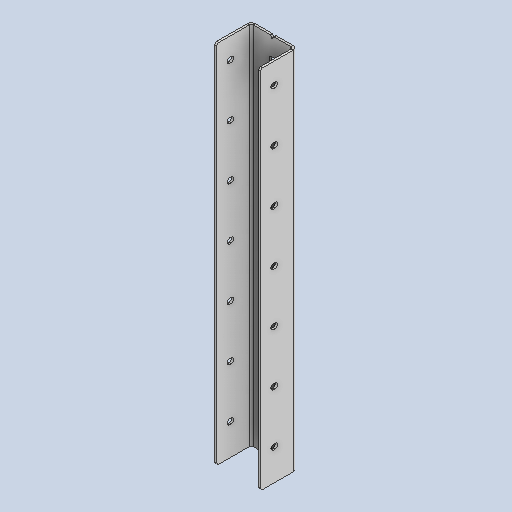
# Autodesk Inventor part: NDM 4.0.1 father bottom
Saved by Autodesk Inventor 2025 (Build 290162010, 162A)
## iProperties
Created: 2023-07-04
Part Number: NDM 4.0.1 father bottom
Material: Stainless Steel
Document SubType Name: Sheet Metal
Designer: user
Density: 8 g/cm^3
Sheet Metal Rule: Default_mm
Appearance: Default
Flat Pattern Width: 10.7048 cm
Flat Pattern Length: 35 cm
Flat Pattern Area: 374.667 cm^2
Sheet Metal Width: 107,048 mm
Sheet Metal Length: 350,000 mm
Sheet Metal Area: 37466,725 mm^2
Stock Number: NDM 7.1 папа ноги домкрат
Description: 2mm
Mass: 592.546 g
Surface Area: 766.755 cm^2
Volume: 74.0682 cm^3
Author: user
Revision Number: 8
Autodesk Inventor part; units mm, degrees
ref_plane "YZ Plane" through (0, 0, 0) normal (1, 0, 0) x (0, 1, 0)
ref_plane "XZ Plane" through (0, 0, 0) normal (0, 1, 0) x (-1, 0, 0)
ref_plane "XY Plane" through (0, 0, 0) normal (0, 0, 1) x (1, 0, 0)
sketch "Sketch1" plane through (0, 0, 0) normal (0, 0, 1) x (1, 0, 0)
  line L0 (-20, 175) -> (20, 175)
  line L1 (20, 175) -> (20, -175)
  line L2 (20, -175) -> (-20, -175)
  line L3 (-20, -175) -> (-20, 175)
  line L4 (-20, 175) -> (20, -175) construction
  line L5 (20, 175) -> (-20, -175) construction
  point P0 (0, 0)
  point P1 (0, 0)
  dimension "d0" = 40
  dimension "d1" = 350
  constraints: 12 end point, 2 midpoint, 1 coincident, 1 horizontal, 1 parallel, 1 perpendicular
  measures "d0" distance of L1.end L2.end
  measures "d1" distance of L2.end L0.start
extrude "Plate1" add sketch "Sketch1" along normal blind 2
sketch "Sketch2" plane through (-20, -175, 2) normal (-1, 0, 0) x (0, -1, 0)
  line L0 (-350, 0) -> (0, 0)
  line L1 (0, 0) -> (0, 33)
  line L2 (0, 33) -> (-350, 33)
  line L3 (-350, 33) -> (-350, 0)
  constraints: 6 end point, 1 horizontal, 1 perpendicular, 1 vertical
edge flange "Flange1" height 35 angle 90 thickness 2 bend radius 2 thickness toward (-1, 0, 0) relief tear relief width 2 relief depth 1 corner gap 2 corner form 0 edges at (-20, 0, 2) (20, 0, 2) wall of the first edge with corners at (-20, 175, 2) (-20, -175, 2) (-20, -175, 35) (-20, 175, 35)
bend "Bend1"
corner "Corner1"
sketch "Sketch3" plane through (0, 0, 0) normal (1, 0, 0) x (0, 1, 0)
  line L0 (-175, 4) -> (175, 4) projected
  line L1 (175, 35) -> (175, 4) projected
  line L2 (-175, 35) -> (175, 35) projected
  line L3 (-175, 4) -> (-175, 35) projected
  circle A0 centre (-145, 22) radius 2.5
  line L4 (-145, 22.75) -> (-145, 21.25) construction
  line L5 (-147.5, 22.75) -> (-147.5, 21.25)
  line L6 (-142.5, 21.25) -> (-142.5, 22.75)
  arc A1 (-142.5, 22.75) -> (-147.5, 22.75) centre (-145, 22.75) ccw
  arc A2 (-147.5, 21.25) -> (-142.5, 21.25) centre (-145, 21.25) ccw
  point P0 (0, 0)
  point P1 (-142.5, 22)
  point P2 (-147.5, 22)
  dimension "d13" = 5
  dimension "d14" = 13
  dimension "d15" = 30
  dimension "d29" = 1.5
  constraints: 8 end point, 5 tangent, 4 point on circle, 3 centre point, 1 coincident, 1 midpoint, 1 parallel, 1 vertical
  measures "d13" diameter of A0
  measures "d14" distance from line of A0.centre L2
  measures "d15" distance from line of L3 A0.centre
  measures "d29" distance of L4.start L4.end
extrude "Extrusion1" cut sketch "Sketch3" along normal through all both and the other way through all contours A0 | L6 A2 L5 A0 | A0 L5 A1 L6
sketch "Sketch4" plane through (0, 0, 0) normal (0, 0, -1) x (-1, 0, 0)
  circle A0 centre (0, -145) radius 2.5
  line L0 (-18, -175) -> (18, -175) projected
  line L1 (-0.5, -145) -> (0.5, -145) construction
  line L2 (-0.5, -147.5) -> (0.5, -147.5)
  line L3 (0.5, -142.5) -> (-0.5, -142.5)
  arc A1 (-0.5, -142.5) -> (-0.5, -147.5) centre (-0.5, -145) ccw
  arc A2 (0.5, -147.5) -> (0.5, -142.5) centre (0.5, -145) ccw
  point P0 (0, 0)
  point P1 (0, -175)
  point P2 (18, -175)
  point P3 (0, -142.5)
  point P4 (0, -147.5)
  dimension "d21" = 5
  dimension "d22" = 30
  dimension "d28" = 1
  constraints: 8 end point, 5 tangent, 4 point on circle, 3 centre point, 1 coincident, 1 horizontal, 1 midpoint, 1 parallel, 1 vertical alignment, 2 other
  measures "d21" diameter of A0
  measures "d28" distance of L1.start L1.end
extrude "Extrusion2" cut sketch "Sketch4" against normal through all
pattern_linear "Rectangular Pattern2" count 7 spacing 50 along (0, 1, 0) of "Extrusion2", "Extrusion1"
fillet "Fillet1" radius 2 4 edges at (-21, -175, 35) (21, -175, 35) (-21, 175, 35) (21, 175, 35)
sketch "Sketch5" plane through (0, 0, 2) normal (0, 0, 1) x (1, 0, 0)
  line L0 (-18, 175) -> (18, 175) projected
  line L1 (-1.5, 175) -> (0, 172)
  line L2 (0, 172) -> (1.5, 175)
  point P0 (0, 0)
  point P1 (0, 175)
  dimension "d31" = 3
  dimension "d32" = 3
  constraints: 4 end point, 2 point on line, 1 equal length, 1 midpoint, 1 vertical alignment
  measures "d31" distance of L2.end L1.start
  measures "d32" distance from line of L1.end L0
extrude "Extrusion3" cut sketch "Sketch5" against normal through all
fillet "Fillet2" radius 0.5 3 edges at (-1.5, 175, 1) (0, 172, 1) (1.5, 175, 1)
mirror "Mirror1" about plane through (0, 0, 0) normal (0, 1, 0) of "Extrusion3"
equation "\"d2\" = Thickness"
equation "\"d3\" = BendReliefWidth"
equation "\"d4\" = BendReliefDepth"
equation "\"d5\" = MinimumRemnant"
equation "\"d6\" = TransitionRadius"
equation "\"d9\" = BendRadius"
equation "\"d10\" = CornerReliefSize"
equation "\"d11\" = GapSize"
equation "\"d12\" = JacobiRadiusSize"
equation "\"BendRadius\" = Thickness"
equation "\"BendReliefWidth\" = Thickness"
equation "\"BendReliefDepth\" = 0.5 * Thickness"
equation "\"CornerReliefSize\" = 4 * Thickness"
equation "\"MinimumRemnant\" = 2 * Thickness"
equation "\"TransitionRadius\" = BendRadius"
equation "\"JacobiRadiusSize\" = BendRadius"
equation "\"GapSize\" = Thickness"
equation "\"Thickness\" = 2"
body "Solid1"
